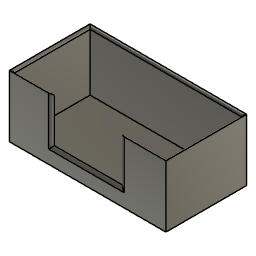
thelio-io-holder-v1 (Autodesk Fusion 360 design; units mm, degrees)
Autodesk Fusion 360 part; units mm, degrees
sketch "Sketch1" plane through (0, 0, 0) normal (0, 0, 1) x (1, 0, 0)
  line L0 (-200, 150) -> (-134, 150)
  line L1 (-134, 150) -> (-134, 116)
  line L2 (-134, 116) -> (-200, 116)
  line L3 (-200, 116) -> (-200, 150)
  dimension "d1" = 66
  dimension "d2" = 34
  constraint horizontal L0
  constraint vertical L1
  constraint horizontal L2
  constraint vertical L3
  measures "d1" distance of L0.start L0.end
  measures "d2" distance of L0.start L2.end
extrude "Extrude1" add sketch "Sketch1" along normal blind 26
shell "Shell1" thickness 1 removed faces 1 at (-178, 138.6667, 26)
sketch "Sketch2" plane through (0, 116, 0) normal (0, -1, 0) x (1, 0, 0)
  line L0 (-200, 0) -> (-134, 0)
  line L1 (-134, 0) -> (-134, 26)
  line L2 (-134, 26) -> (-200, 26)
  line L3 (-200, 26) -> (-200, 0)
  line L4 (-182.0469, 26) -> (-182.0469, 7)
  line L5 (-182.0469, 7) -> (-153, 7)
  line L6 (-153, 7) -> (-153, 26)
  constraint coincident L2 L4.start
  constraint perpendicular L2 L4
  constraint perpendicular L4 L5
  constraint coincident L2 L6.end
  constraint perpendicular L2 L6
extrude "Extrude2" cut sketch "Sketch2" against normal blind 3 contours L2 L4 L5 L6
fillet "Fillet1" radius 1.5 3 edges at (-182.0469, 116, 16.5) (-167.5235, 116, 7) (-153, 116, 16.5)
fillet "Fillet2" radius 1 5 edges at (-199, 133, 26) (-167, 149, 26) (-135, 133, 26) (-144, 117, 26) (-190.5235, 117, 26)
